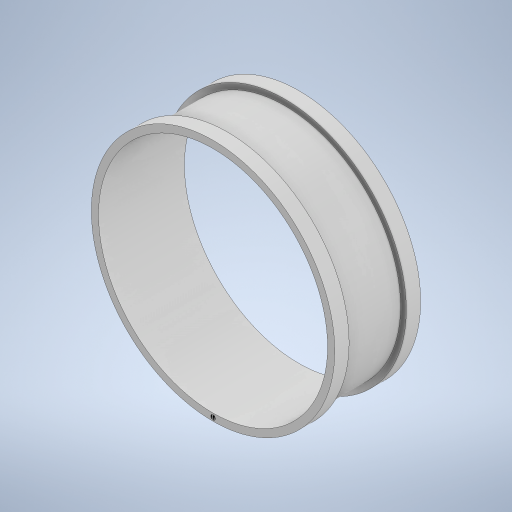
# Autodesk Inventor part: In1
Saved by Autodesk Inventor 2023 (Build 270158000, 158)
## iProperties
Created: 2023-10-09
Part Number: In1
Material: Generic
Document SubType Name: Modeling
Designer: huy20
Density: 1 g/cm^3
Appearance: Default
Author: huy20
Autodesk Inventor part; units mm, degrees
ref_plane "YZ Plane" through (0, 0, 0) normal (1, 0, 0) x (0, 1, 0)
ref_plane "XZ Plane" through (0, 0, 0) normal (0, 1, 0) x (-1, 0, 0)
ref_plane "XY Plane" through (0, 0, 0) normal (0, 0, 1) x (1, 0, 0)
sketch "Sketch1" plane through (0, 0, 0) normal (0, 0, 1) x (1, 0, 0)
  circle A0 centre (0, 0) radius 4
  circle A1 centre (0, 0) radius 4.25
  dimension "d0" = 8
  dimension "d1" = 8.5
  constraints: 2 centre point, 2 coincident
  measures "d0" diameter of A0
  measures "d1" diameter of A1
extrude "Extrusion1" add sketch "Sketch1" along normal mid plane 3
sketch "Sketch5" plane through (0, 0, 0) normal (0, 1, 0) x (-1, 0, 0)
  line L0 (0, -2.1235) -> (0, 2.5622)
  line L1 (4.25, -1.5) -> (4.25, 1.5) projected
  line L2 (4.25, -1) -> (4.05, -1)
  line L3 (4.05, -1) -> (4.05, 1)
  line L4 (4.05, 1) -> (4.25, 1)
  line L5 (-4.25, -1.5) -> (4.25, -1.5) projected
  point P0 (0, 0)
  dimension "d12" = 0.2
  dimension "d13" = 2
  dimension "d14" = 0.5
  constraints: 8 end point, 3 perpendicular, 2 point on line, 1 vertical
  measures "d12" distance between parallel lines of L1 L3
  measures "d13" distance of L2.end L3.end
  measures "d14" distance between parallel lines of L2 L5
revolve "Revolution1" cut sketch "Sketch5" angle 360 about axis through (0, 0, -2.1235) along (0, 0, 1)
sketch "Sketch6" plane through (0, 0, 1.5) normal (0, 0, 1) x (1, 0, 0)
  circle A0 centre (0, -4.1314) radius 0.0831
  point P0 (0, 0)
  constraints: 1 centre point
extrude "Extrusion2" add sketch "Sketch6" against normal blind 0.1 separate body
mirror "Mirror1" about plane through (0, 0, 0) normal (0, 0, 1) of "Extrusion2" bodies 2
body "Solid1"
body "Solid2"
